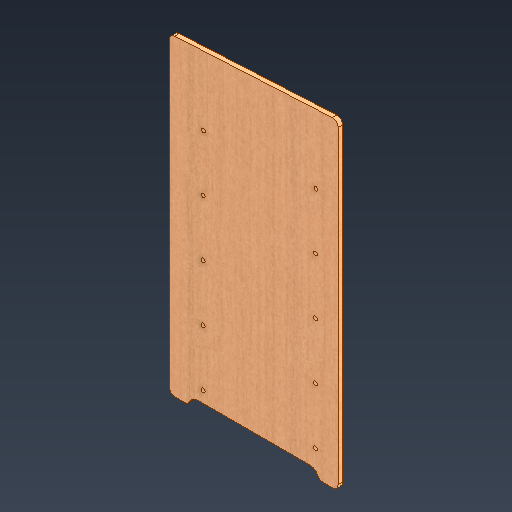
# Autodesk Inventor part: side_panel
Saved by Autodesk Inventor 2021 (Build 250183000, 183)
## iProperties
Created: 2023-03-31
Part Number: side_panel
Material: 木材(サクラ)
Document SubType Name: Modeling
Designer: casey
Density: 0.63 g/cm^3
Appearance: サクラ材 - ナチュラル 抑えた光沢
Author: casey
Autodesk Inventor part; units mm, degrees
ref_plane "YZ Plane" through (0, 0, 0) normal (1, 0, 0) x (0, 1, 0)
ref_plane "XZ Plane" through (0, 0, 0) normal (0, 1, 0) x (-1, 0, 0)
ref_plane "XY Plane" through (0, 0, 0) normal (0, 0, 1) x (1, 0, 0)
sketch "スケッチ1" plane through (0, 0, 0) normal (0, 0, 1) x (1, 0, 0)
  line L0 (0, 0) -> (150, 0)
  line L1 (150, 0) -> (150, -300)
  line L2 (150, -300) -> (0, -300)
  line L3 (0, -300) -> (0, 0)
  line L4 (150, -15) -> (0, -22.8612)
  circle A0 centre (130.1882, -77.2664) radius 1.75 projected
  circle A1 centre (30.3252, -82.5) radius 1.75 projected
  line L5 (130.1882, -77.2664) -> (30.3252, -82.5)
  dimension "d2" = 150
  dimension "d3" = 300
  dimension "d68" = 15
  constraints: 12 end point, 3 parallel, 2 point on line, 1 horizontal, 1 perpendicular
  measures "d2" distance of L1.end L2.end
  measures "d3" distance of L0.end L1.end
  measures "d68" distance from line of L4.start L0
extrude "押し出し1" add sketch "スケッチ1" along normal blind 4 contours L4 L1 L2 L3 | A0 | A1
sketch "スケッチ2" plane through (0, 0, 0) normal (0, 0, -1) x (-1, 0, 0)
  line L0 (-125, -300) -> (-25, -300) construction
  line L1 (0, -300) -> (-150, -300) projected
  line L2 (-125, -307.5) -> (-25, -307.5)
  line L3 (-25, -292.5) -> (-125, -292.5)
  arc A0 (-125, -292.5) -> (-125, -307.5) centre (-125, -300) ccw
  arc A1 (-25, -307.5) -> (-25, -292.5) centre (-25, -300) ccw
  point P0 (0, 0)
  point P1 (-75, -300)
  point P2 (-132.5, -300)
  point P3 (-17.5, -300)
  dimension "d4" = 50
  dimension "d5" = 15
  constraints: 8 end point, 4 point on circle, 4 tangent, 2 centre point, 2 midpoint, 1 parallel, 1 point on line
  measures "d4" distance of point (-75, -300) L0.end
  measures "d5" diameter of A1
extrude "押し出し2" cut sketch "スケッチ2" against normal blind 4 contours L1 A0 L3 A1
fillet "フィレット1" radius 5 4 edges at (150, -300, 2) (132.5, -300, 2) (17.5, -300, 2) (0, -300, 2)
sketch "スケッチ3" plane through (0, 0, 0) normal (0, 0, -1) x (-1, 0, 0)
  line L0 (0, 0) -> (0, -295) projected
  line L1 (-125, -292.5) -> (-25, -292.5) projected
  line L2 (-129.863, -277.2664) -> (-30, -282.5)
  line L3 (-129.9354, -127.2664) -> (-30.0724, -132.5)
  line L4 (-129.884, -177.2664) -> (-30.021, -182.5)
  line L5 (-130.1882, -77.2664) -> (-30.3252, -82.5)
  line L6 (-150, 0) -> (0, 0) projected
  line L7 (-129.863, -227.2664) -> (-30, -232.5)
  dimension "d16" = 30
  dimension "d17" = 10
  dimension "d18" = 100
  dimension "d19" = 3
  dimension "d61" = 50
  dimension "d65" = 50
  dimension "d66" = 50
  dimension "d67" = 50
  constraints: 10 end point, 8 parallel
  measures "d16" distance from line of L0 L2.end
  measures "d17" distance from line of L1 L2.end
  measures "d18" distance of L2.start L2.end
  measures "d19" angle of L1 L2
  measures "d61" distance of L2.end L7.end
  measures "d65" distance of L4.end L7.end
  measures "d66" distance of L3.end L4.end
  measures "d67" vertical distance of L5.end L3.end
hole "穴1" at (30, -282.5, 0) at (129.863, -277.2664, 0) at (129.863, -227.2664, 0) at (129.9354, -127.2664, 0) at (30.0724, -132.5, 0) at (129.884, -177.2664, 0) at (30.021, -182.5, 0) at (130.1882, -77.2664, 0) at (30.3252, -82.5, 0) at (30, -232.5, 0) direction (0, 0, 1) diameter 3.5 end through all
fillet "フィレット2" radius 5 2 edges at (150, -15, 2) (0, -22.8612, 2)
